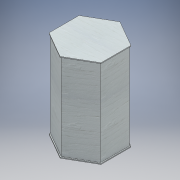
# Autodesk Inventor part: Hexagono
Saved by Autodesk Inventor 2017 (Build 210142000, 142)
## iProperties
Created: 2016-07-03
Part Number: Hexagono
Material: Generic
Document SubType Name: Modeling
Designer: Ing
Density: 1 g/cm^3
Appearance: Default
Author: Ing
Autodesk Inventor part; units mm, degrees
ref_plane "YZ Plane" through (0, 0, 0) normal (1, 0, 0) x (0, 1, 0)
ref_plane "XZ Plane" through (0, 0, 0) normal (0, 1, 0) x (-1, 0, 0)
ref_plane "XY Plane" through (0, 0, 0) normal (0, 0, 1) x (1, 0, 0)
sketch "Sketch1" plane through (0, 0, 0) normal (0, 0, 1) x (1, 0, 0)
  line L0 (0, 50) -> (43.3013, 25)
  line L1 (43.3013, 25) -> (43.3013, -25)
  line L2 (43.3013, -25) -> (0, -50)
  line L3 (0, -50) -> (-43.3013, -25)
  line L4 (-43.3013, -25) -> (-43.3013, 25)
  line L5 (-43.3013, 25) -> (0, 50)
  line L6 (-43.3013, 0) -> (-41.8013, 0)
  line L7 (-41.8013, 0) -> (-41.8013, 19.6162)
  line L8 (-41.8013, 0) -> (-41.8013, -22.4019)
  line L9 (-41.8013, 24.1299) -> (-0.0035, 48.2659)
  line L10 (-0.0035, 48.2659) -> (41.7978, 24.136)
  line L11 (41.7978, 24.136) -> (41.8013, -24.1299)
  line L12 (41.8013, -24.1299) -> (0.0035, -48.2659)
  line L13 (0.0035, -48.2659) -> (-41.7978, -24.136)
  line L14 (-41.7978, -24.136) -> (-41.8013, 24.1299)
  point P0 (0, 0)
  point P1 (41.8008, -18.0468)
  point P2 (43.3013, -18.0468)
  point P3 (41.8009, -18.3387)
  point P4 (43.3013, -18.3387)
  dimension "d0" = 50
  dimension "d11" = 1.5
  dimension "d12" = 0.004
  dimension "d13" = 1.5004
  constraints: 30 end point, 5 point on line, 1 horizontal, 1 midpoint, 1 perpendicular, 1 vertical, 13 other
  measures "d0" distance of L3.end L4.end
  measures "d11" distance of L6.start L6.end
  measures "d12" angle of L13 L3
  measures "d13" distance from line of point (43.301, -18.339) L11
extrude "Extrusion3" add sketch "Sketch1" along normal blind 150
sketch "Sketch2" plane through (0, 0, 150) normal (0, 0, 1) x (1, 0, 0)
  line L0 (0, 0) -> (0, 52)
  line L1 (0, 52) -> (45.0333, 26)
  line L2 (45.0333, 26) -> (45.0333, -26)
  line L3 (45.0333, -26) -> (0, -52)
  line L4 (0, -52) -> (-45.0333, -26)
  line L5 (-45.0333, -26) -> (-45.0333, 26)
  line L6 (-45.0333, 26) -> (0, 52)
  dimension "d16" = 52
  dimension "d17" = 52
  constraints: 14 end point, 1 coincident, 1 vertical, 13 other
  measures "d16" distance of L4.end L5.end
  measures "d17" distance of L1.end L2.end
extrude "Extrusion4" add sketch "Sketch2" along normal blind 1.5
sketch "Sketch3" plane through (0, 0, 0) normal (0, 0, -1) x (-1, 0, 0)
  line L0 (45.0333, -26) -> (0, -52) projected
  line L1 (0, -52) -> (-45.0333, -26)
  line L2 (-45.0333, -26) -> (-45.0333, 26)
  line L3 (-45.0333, 26) -> (0, 52)
  line L4 (0, 52) -> (45.0333, 26)
  line L5 (45.0333, 26) -> (45.0333, -26)
  line L6 (45.0333, -26) -> (0, -52)
  point P0 (0, 0)
  point P1 (0, 0)
  dimension "d20" = 52
  constraints: 12 end point, 1 coincident, 13 other
  measures "d20" distance of L4.end L5.end
extrude "Extrusion5" add sketch "Sketch3" along normal blind 1.5
body "Solid3"
